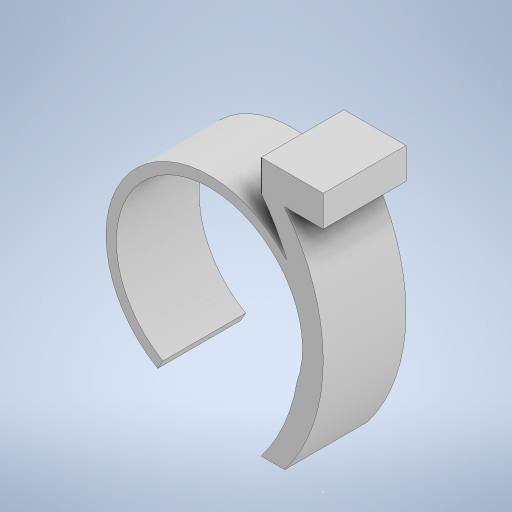
# Autodesk Inventor part: tetik2
Saved by Autodesk Inventor 2023 (Build 270158000, 158)
## iProperties
Created: 2023-02-01
Part Number: tetik2
Material: Generic
Document SubType Name: Modeling
Designer: Umut Yücesoy
Density: 1 g/cm^3
Appearance: Default
Author: Umut Yücesoy
Autodesk Inventor part; units mm, degrees
ref_plane "YZ Plane" through (0, 0, 0) normal (1, 0, 0) x (0, 1, 0)
ref_plane "XZ Plane" through (0, 0, 0) normal (0, 1, 0) x (-1, 0, 0)
ref_plane "XY Plane" through (0, 0, 0) normal (0, 0, 1) x (1, 0, 0)
sketch "Sketch1" plane through (0, 0, 0) normal (0, 1, 0) x (-1, 0, 0)
  line L0 (0, 0) -> (6, 0)
  line L1 (6, 0) -> (6, -8)
  line L2 (6, -8) -> (0, -8)
  line L3 (0, -8) -> (0, 0)
  dimension "d0" = 6
  dimension "d1" = 8
  constraints: 8 end point, 2 parallel, 1 horizontal, 1 perpendicular
  measures "d0" distance of L1.end L2.end
  measures "d1" distance of L0.end L1.end
extrude "Extrusion1" add sketch "Sketch1" along normal blind 25
sketch "Sketch5" plane through (-6, 0, 0) normal (0, 0, 1) x (1, 0, 0)
  line L0 (0, 0) -> (0, 25) projected
  line L1 (0, 0) -> (-30, 0)
  line L2 (-30, 0) -> (-30, 25)
  line L3 (-30, 25) -> (0, 25)
  line L4 (0, 25) -> (0, 0)
  point P0 (6, 0)
  dimension "d9" = 30
  constraints: 8 end point, 2 parallel, 1 horizontal, 1 perpendicular
  measures "d9" distance of L2.end L3.end
extrude "Extrusion4" add sketch "Sketch5" against normal blind 25
sketch "Sketch6" plane through (0, 0, 0) normal (0, 0, 1) x (1, 0, 0)
  line L0 (0, 0) -> (-6, 0) projected
  line L1 (-6, 0) -> (-6, 25) projected
  line L2 (0, 25) -> (-6, 25) projected
  line L3 (0, 0) -> (0, 25) projected
  line L4 (-6, 25) -> (-6, 0) projected
  line L5 (0, 0) -> (-6, 0) projected
  line L6 (-6, 0) -> (-6, 25) projected
  line L7 (0, 25) -> (-6, 25) projected
  line L8 (0, 0) -> (0, 25) projected
  line L9 (0, 0) -> (0, 25) projected
  line L10 (0, 25) -> (0, 22)
  line L11 (0, 22) -> (-36, 22)
  line L12 (-36, 0) -> (-36, 25) projected
  circle A0 centre (-11, 11) radius 10
  arc A1 (-6, 0) -> (-6, 22) centre (-20.3784, 11) ccw
  arc A2 (-3.7301, 0) -> (-3.7301, 22) centre (-18.1085, 11) ccw
  circle A3 centre (-11, 11) radius 9
  line L13 (-11, 11) -> (-18, -1.1244)
  line L14 (-11, 11) -> (3, 11) construction
  line L15 (0, 22) -> (0, 0)
  line L16 (-36, 0) -> (0, 0) projected
  line L17 (-3.7301, 0) -> (0, 0)
  line L18 (-17.3509, 0) -> (-36, 0)
  line L19 (-36, 0) -> (-36, 25)
  line L20 (-6, 25) -> (-6, 22)
  point P0 (-2.5346, 7.9443)
  point P1 (-15.5, 3.2058)
  point P2 (-16, 2.3397)
  point P3 (-3.5476, 17.6679)
  dimension "d12" = 3
  dimension "d13" = 20
  dimension "d14" = 18
  dimension "d15" = 120
  constraints: 18 end point, 6 point on line, 4 centre point, 4 point on circle, 3 collinear, 2 horizontal, 2 perpendicular, 1 coincident, 1 equal length
  measures "d12" distance of L2.start L10.end
  measures "d13" diameter of A0
  measures "d14" diameter of A3
  measures "d15" angle of L13 L14
extrude "Extrusion5" cut sketch "Sketch6" against normal blind 25 contours L16 L13 A0 L1 | L1 A0 A1 | A0 L13 A3 L1 | L1 A3 A1 A0 | L16 L12 L11 L1 A0 L13 | A1 A0 L1 | A3 L1 | L1 A3 A1 | A1 A3 picked at (-6.5916, 2.8181) picked at (-4.9439, 3.9447)
sketch "Sketch7" plane through (0, 0, 0) normal (0, 0, 1) x (1, 0, 0)
  line L0 (-6, 22) -> (-6, 25) projected
  line L1 (-6, 22) -> (-6, 25)
  point P0 (0, 0)
  constraints: 2 end point, 1 collinear
sketch "Sketch9" plane through (-6, 25, -8) normal (1, 0, 0) x (0, 0, -1)
  line L0 (0, -25) -> (0, 0) projected
  line L1 (0, 0) -> (18.2741, 0)
  line L2 (18.2741, 0) -> (18.2741, -25.5609)
  line L3 (18.2741, -25.5609) -> (0, -25.5609)
  line L4 (0, -25.5609) -> (0, 0)
  point P0 (-8, -25)
  constraints: 8 end point, 2 parallel, 1 horizontal, 1 perpendicular
extrude "Extrusion6" cut sketch "Sketch9" against normal blind 39.25
sketch "Sketch11" plane through (0, 0, -8) normal (0, 0, -1) x (-1, 0, 0)
  line L0 (36, 22) -> (6, 22) projected
  line L1 (36, 25) -> (36, 22) projected
  line L2 (6, 22) -> (36, 22)
  line L3 (36, 22) -> (36, 25)
  line L4 (36, 25) -> (6, 25)
  line L5 (6, 25) -> (6, 22)
  point P0 (0, 0)
  constraints: 8 end point, 2 parallel, 1 horizontal, 1 perpendicular
extrude "Extrusion8" cut sketch "Sketch11" against normal blind 39.25
sketch "Sketch12" plane through (0, 0, 0) normal (0, 0, 1) x (1, 0, 0)
  line L0 (0, 0) -> (-6, 0) projected
  arc A0 (-3.5476, 17.6679) -> (-6, 22) centre (-20.3784, 11) ccw projected
  arc A1 (-3.7251, 0) -> (-3.7281, 22) centre (-18.105, 10.9981) ccw
  line L1 (-3.7281, 22) -> (0, 22)
  line L2 (0, 0) -> (0, 25) projected
  line L3 (0, 22) -> (0, 0)
  line L4 (0, 0) -> (-3.7251, 0)
  point P0 (0, 22)
  point P1 (-3.7251, 0)
  constraints: 6 end point, 2 perpendicular, 2 point on circle, 1 centre point, 1 horizontal
extrude "Extrusion9" cut sketch "Sketch12" against normal blind 39.25
body "Solid1"
